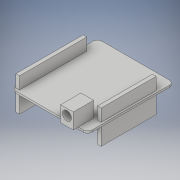
# Autodesk Inventor part: board_mockup
Saved by Autodesk Inventor 2017 (Build 210142000, 142)
## iProperties
Created: 2018-05-31
Part Number: board_mockup
Material: Generic
Document SubType Name: Modeling
Designer: sinner
Density: 1 g/cm^3
Appearance: Default
Author: sinner
Autodesk Inventor part; units mm, degrees
ref_plane "YZ Plane" through (0, 0, 0) normal (1, 0, 0) x (0, 1, 0)
ref_plane "XZ Plane" through (0, 0, 0) normal (0, 1, 0) x (-1, 0, 0)
ref_plane "XY Plane" through (0, 0, 0) normal (0, 0, 1) x (1, 0, 0)
sketch "Sketch1" plane through (0, 0, 0) normal (0, 1, 0) x (-1, 0, 0)
  line L0 (0, 0) -> (53.34, 0)
  line L1 (53.34, 0) -> (53.34, -60.2234)
  line L2 (53.34, -60.2234) -> (0, -60.2234)
  line L3 (0, -60.2234) -> (0, 0)
  dimension "d0" = 53.34
  dimension "d1" = 60.2234
  constraints: 8 end point, 2 parallel, 1 horizontal, 1 perpendicular
  measures "d0" distance of L1.end L2.end
  measures "d1" distance of L0.end L1.end
extrude "Extrusion1" add sketch "Sketch1" along normal blind 1.397
fillet "Fillet1" radius 3.175 4 edges at (0, 0.6985, -60.2234) (-53.34, 0.6985, -60.2234) (0, 0.6985, 0) (-53.34, 0.6985, 0)
sketch "Sketch2" plane through (0, 1.397, 0) normal (0, 1, 0) x (1, 0, 0)
  line L0 (0, 0) -> (-74.2846, 0) construction
  line L1 (0, 0) -> (0, 92.3898) construction
  line L2 (-3.9116, 10.795) -> (-1.3716, 10.795)
  line L3 (-1.3716, 10.795) -> (-1.3716, 49.2506)
  line L4 (-1.3716, 49.2506) -> (-3.9116, 49.2506)
  line L5 (-3.9116, 49.2506) -> (-3.9116, 10.795)
  line L6 (-51.9684, 1.778) -> (-49.4284, 1.778)
  line L7 (-49.4284, 1.778) -> (-49.4284, 48.8569)
  line L8 (-49.4284, 48.8569) -> (-51.9684, 48.8569)
  line L9 (-51.9684, 48.8569) -> (-51.9684, 1.778)
  line L10 (-53.34, 57.0484) -> (-53.34, 3.175) projected
  line L11 (-53.34, 50.5823) -> (-53.34, -10.1143) construction
  dimension "d5" = 2.54
  dimension "d6" = 2.54
  dimension "d7" = 38.4556
  dimension "d8" = 47.0789
  dimension "d9" = 1.778
  dimension "d10" = 3.9116
  dimension "d11" = 10.795
  dimension "d12" = 3.9116
  constraints: 22 end point, 4 parallel, 3 horizontal, 2 perpendicular, 1 collinear, 1 point on line, 1 vertical
  measures "d5" distance of L7.end L8.end
  measures "d6" distance of L3.end L4.end
  measures "d7" distance of L4.end L2.start
  measures "d8" distance of L6.end L7.end
  measures "d9" distance between parallel lines of L0 L6
  measures "d10" distance between parallel lines of L10 L7
  measures "d11" distance between parallel lines of L0 L2
  measures "d12" distance between parallel lines of L1 L5
extrude "Extrusion2" add sketch "Sketch2" along normal blind 8.636
sketch "Sketch3" plane through (0, 1.397, 0) normal (0, 1, 0) x (1, 0, 0)
  line L0 (0, 0) -> (-18.0314, 0) construction
  line L1 (-50.165, 0) -> (-3.175, 0) projected
  line L2 (0, 0) -> (0, 13.9144) construction
  line L3 (0, 3.175) -> (0, 57.0484) projected
  line L4 (-15.3162, -3.556) -> (-6.477, -3.556)
  line L5 (-6.477, -3.556) -> (-6.477, 10.668)
  line L6 (-6.477, 10.668) -> (-15.3162, 10.668)
  line L7 (-15.3162, 10.668) -> (-15.3162, -3.556)
  dimension "d19" = 8.8392
  dimension "d20" = 14.224
  dimension "d21" = 3.556
  dimension "d22" = 6.477
  constraints: 12 end point, 2 parallel, 2 point on line, 1 horizontal, 1 perpendicular
  measures "d19" distance of L5.end L6.end
  measures "d20" distance of L6.end L4.start
  measures "d21" distance between parallel lines of L0 L4
  measures "d22" distance between parallel lines of L2 L5
extrude "Extrusion3" add sketch "Sketch3" along normal blind 10.8839
sketch "Sketch4" plane through (0, 0, 0) normal (0, -1, 0) x (1, 0, 0)
  line L0 (0, 0) -> (0, -16.5285) construction
  line L1 (0, -3.175) -> (0, -57.0484) projected
  line L2 (0, 0) -> (-10.3791, 0) construction
  line L3 (-3.175, 0) -> (-50.165, 0) projected
  line L4 (-49.4284, -48.8569) -> (-49.4284, -1.778) projected
  line L5 (-51.9684, -1.778) -> (-51.9684, -48.8569) projected
  line L6 (-49.4284, -1.778) -> (-51.9684, -1.778)
  line L7 (-51.9684, -1.778) -> (-51.9684, -48.8569)
  line L8 (-51.9684, -48.8569) -> (-49.4284, -48.8569)
  line L9 (-49.4284, -48.8569) -> (-49.4284, -1.778)
  line L10 (-1.3716, -10.795) -> (-3.9116, -10.795)
  line L11 (-3.9116, -10.795) -> (-3.9116, -49.2506)
  line L12 (-3.9116, -49.2506) -> (-1.3716, -49.2506)
  line L13 (-1.3716, -49.2506) -> (-1.3716, -10.795)
  dimension "d25" = 47.0789
  dimension "d27" = 2.54
  dimension "d28" = 38.4556
  dimension "d29" = 10.795
  dimension "d30" = 3.9116
  dimension "d31" = 1.778
  constraints: 20 end point, 4 parallel, 4 point on line, 2 horizontal, 2 perpendicular
  measures "d25" distance of L8.end L6.start
  measures "d27" distance of L11.end L12.end
  measures "d28" distance of L12.end L10.start
  measures "d29" distance between parallel lines of L3 L10
  measures "d30" distance between parallel lines of L1 L11
  measures "d31" distance between parallel lines of L3 L6
extrude "Extrusion4" add sketch "Sketch4" along normal blind 13.1572
sketch "Sketch5" plane through (-15.3162, 1.397, 3.556) normal (0, 0, 1) x (1, 0, 0)
  circle A0 centre (4.4196, 6.4389) radius 3.175
  line L0 (0, 10.8839) -> (8.8392, 10.8839) projected
  line L1 (4.4196, 10.8839) -> (4.4196, -0.1131) construction
  point P0 (15.3162, -1.397)
  dimension "d34" = 6.35
  dimension "d35" = 4.445
  constraints: 2 end point, 1 centre point, 1 midpoint, 1 point on line, 1 vertical
  measures "d34" diameter of A0
  measures "d35" distance from line of L0 A0.centre
extrude "Extrusion5" cut sketch "Sketch5" against normal blind 6.35
body "Solid1"
